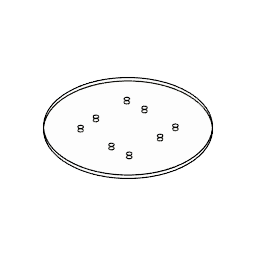
LowerPlate_v12 (Autodesk Fusion 360 design; units mm, degrees)
Autodesk Fusion 360 part; units mm, degrees
sketch "Sketch1" plane through (0, 0, 0) normal (0, 0, 1) x (1, 0, 0)
  circle A0 centre (0, 0) radius 60
  line L0 (-36.4192, 17.7153) -> (3.5808, 17.7153)
  line L1 (3.5808, 17.7153) -> (3.5808, -2.2847)
  line L2 (3.5808, -2.2847) -> (-36.4192, -2.2847)
  line L3 (-36.4192, -2.2847) -> (-36.4192, 17.7153)
  line L4 (-17.7153, -36.4192) -> (-17.7153, 3.5808)
  line L5 (-17.7153, 3.5808) -> (2.2847, 3.5808)
  line L6 (2.2847, 3.5808) -> (2.2847, -36.4192)
  line L7 (2.2847, -36.4192) -> (-17.7153, -36.4192)
  line L8 (36.4192, -17.7153) -> (-3.5808, -17.7153)
  line L9 (-3.5808, -17.7153) -> (-3.5808, 2.2847)
  line L10 (-3.5808, 2.2847) -> (36.4192, 2.2847)
  line L11 (36.4192, 2.2847) -> (36.4192, -17.7153)
  line L12 (17.7153, 36.4192) -> (17.7153, -3.5808)
  line L13 (17.7153, -3.5808) -> (-2.2847, -3.5808)
  line L14 (-2.2847, -3.5808) -> (-2.2847, 36.4192)
  line L15 (-2.2847, 36.4192) -> (17.7153, 36.4192)
  line L16 (-24.4192, 23.2153) -> (-24.4192, -7.7847) construction
  line L17 (-36.4192, 7.7153) -> (-24.4192, 7.7153) construction
  circle A1 centre (-24.4192, 23.2153) radius 2
  circle A2 centre (-24.4192, -7.7847) radius 2
  circle A3 centre (7.7847, -24.4192) radius 2
  circle A4 centre (-23.2153, -24.4192) radius 2
  circle A5 centre (24.4192, 7.7847) radius 2
  circle A6 centre (24.4192, -23.2153) radius 2
  circle A7 centre (-7.7847, 24.4192) radius 2
  circle A8 centre (23.2153, 24.4192) radius 2
  line L18 (-36.4192, 7.7153) -> (-50, 7.7153) construction
  line L19 (-50, 19.7153) -> (-50, -4.2847) construction
  circle A9 centre (-50, -4.2847) radius 3
  circle A10 centre (-50, 19.7153) radius 3
  circle A11 centre (-19.7153, -50) radius 3
  circle A12 centre (4.2847, -50) radius 3
  circle A13 centre (50, -19.7153) radius 3
  circle A14 centre (50, 4.2847) radius 3
  circle A15 centre (19.7153, 50) radius 3
  circle A16 centre (-4.2847, 50) radius 3
  point P0 (-24.4192, 7.7153)
  dimension "d1" = 120
  dimension "d2" = 40
  dimension "d3" = 20
  dimension "d6" = 31
  dimension "d7" = 12
  dimension "d8" = 4
  dimension "d9" = 4
  dimension "d16" = 24
  dimension "d17" = 6
  dimension "d18" = 6
  dimension "d20" = 360
  constraint coincident A0.centre origin
  constraint horizontal L0
  constraint vertical L1
  constraint horizontal L2
  constraint vertical L3
  constraint midpoint L16 P0
  constraint perpendicular L2 L16
  constraint midpoint L3 L17.start
  constraint coincident P0 L17.end
  constraint perpendicular L3 L17
  constraint coincident L16.start A1.centre
  constraint coincident L16.end A2.centre
  constraint perpendicular L3 L18
  constraint midpoint L18.end L19
  constraint perpendicular L18 L19
  constraint coincident L19.end A9.centre
  constraint coincident L19.start A10.centre
  measures "d1" diameter of A0
  measures "d2" distance of L0.start L0.end
  measures "d3" distance of L0.start L2.end
  measures "d6" distance of L16.start L16.end
  measures "d7" horizontal distance of L17.start P0
  measures "d8" diameter of A1
  measures "d9" diameter of A2
  measures "d16" distance of L19.start L19.end
  measures "d17" diameter of A9
  measures "d18" diameter of A10
extrude "Extrude1" add sketch "Sketch1" along normal blind 3 contours A0 | L0 L2 L3 L4 L5 L14 | L0 L1 L10 L12 L14 L15 | L0 L1 L5 L6 L10 L14 | L2 L4 L5 L9 L10 L14 | L5 L6 L10 L14 | L2 L4 L6 L7 L8 L9 | L1 L2 L6 L10 L12 L13 | L1 L2 L6 L10 | L2 L9 L10 L14 | L2 L6 L10 L14 | L2 L6 L8 L9 L13 L14 | L6 L8 L10 L11 L12 L13 | L2 L6 L13 L14 | A9 | A10 | A11 | A12 | A13 | A14 | A15 | A16
